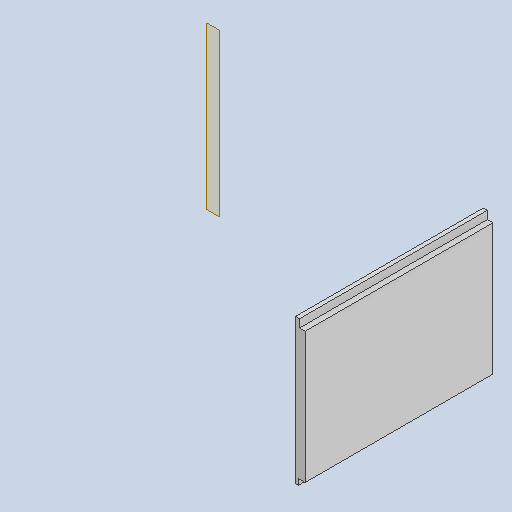
# Autodesk Inventor part: Panel
Saved by Autodesk Inventor 2022 (Build 260153000, 153)
## iProperties
Created: 2021-11-17
Part Number: Panel
Material: Generic
Document SubType Name: Modeling
Designer: Frankie
Density: 1 g/cm^3
Appearance: Default
Author: Frankie
Autodesk Inventor part; units mm, degrees
ref_plane "YZ Plane" through (0, 0, 0) normal (1, 0, 0) x (0, 1, 0)
ref_plane "XZ Plane" through (0, 0, 0) normal (0, 1, 0) x (-1, 0, 0)
ref_plane "XY Plane" through (0, 0, 0) normal (0, 0, 1) x (1, 0, 0)
ref_plane "Work Plane1" through (142.24, 53.9873, -122.2375) normal (0, 0, 1) x (1, 0, 0)
sketch "Sketch1" plane through (142.24, 53.9873, -122.2375) normal (0, 0, 1) x (1, 0, 0)
  line L0 (174.6949, 37.0783) -> (178.6893, 37.0783) projected
  line L1 (174.6949, -58.3128) -> (174.6949, 37.0783) projected
  line L2 (178.0128, -58.3128) -> (174.6949, -58.3128) projected
  line L3 (178.0128, -54.6097) -> (178.0128, -58.3128) projected
  line L4 (182.3149, -54.6097) -> (178.0128, -54.6097) projected
  line L5 (182.3149, 31.8435) -> (182.3149, -54.6097) projected
  line L6 (178.6893, 31.8435) -> (182.3149, 31.8435) projected
  line L7 (178.6893, 37.0783) -> (178.6893, 31.8435) projected
  line L8 (181.6164, -53.9112) -> (177.3143, -53.9112)
  line L9 (177.3143, -53.9112) -> (177.3143, -57.6143)
  line L10 (177.3143, -57.6143) -> (175.3934, -57.6143)
  line L11 (175.3934, -57.6143) -> (175.3934, 36.3798)
  line L12 (175.3934, 36.3798) -> (177.9908, 36.3798)
  line L13 (177.9908, 36.3798) -> (177.9908, 31.145)
  line L14 (177.9908, 31.145) -> (181.6164, 31.145)
  line L15 (181.6164, 31.145) -> (181.6164, -53.9112)
  point P0 (-142.24, -53.9873)
  dimension "d0" = 0.6985
  constraints: 16 end point, 7 other
  measures "d0" distance between parallel lines of L5 L15
extrude "Extrusion1" add sketch "Sketch1" along normal blind 121.92 contours L8 L9 L10 L11 L12 L13 L14 L15
body "Solid1"
